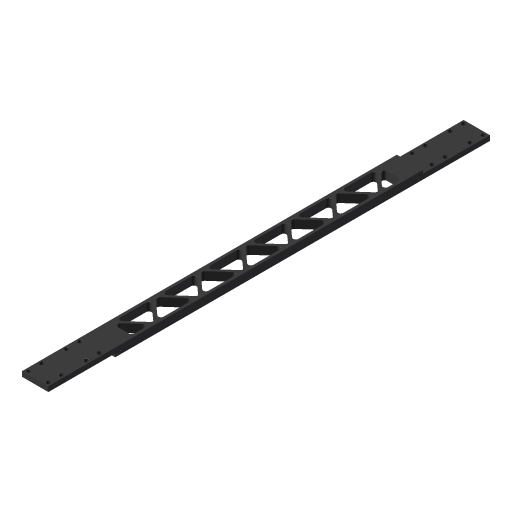
# Autodesk Inventor part: Connector Plate350mm
Saved by Autodesk Inventor 2023 (Build 270158000, 158)
## iProperties
Created: 2022-09-25
Part Number: Connector Plate350mm
Material: Generic
Document SubType Name: Modeling
Designer: deli
Density: 1 g/cm^3
Appearance: Default
Mass: 15.4529 g
Surface Area: 147.421 cm^2
Volume: 15.4529 cm^3
Author: deli
Autodesk Inventor part; units mm, degrees
ref_plane "YZ Plane" through (0, 0, 0) normal (1, 0, 0) x (0, 1, 0)
ref_plane "XZ Plane" through (0, 0, 0) normal (0, 1, 0) x (-1, 0, 0)
ref_plane "XY Plane" through (0, 0, 0) normal (0, 0, 1) x (1, 0, 0)
sketch "Sketch1" plane through (0, 0, 0) normal (0, 1, 0) x (-1, 0, 0)
  line L0 (25.6456, 366.5178) -> (5.6456, 366.5178)
  line L1 (5.6456, 366.5178) -> (5.6456, 30.4178)
  line L2 (5.6456, 30.4178) -> (25.6456, 30.4178)
  line L3 (25.6456, 30.4178) -> (25.6456, 366.5178)
  circle A0 centre (23.1456, 364.0178) radius 1.6
  circle A1 centre (23.1456, 354.0178) radius 1.6
  circle A2 centre (8.1456, 364.0178) radius 1.6
  circle A3 centre (8.1456, 354.0178) radius 1.6
  line L4 (23.1456, 364.0178) -> (23.1456, 354.0178) construction
  line L5 (23.1456, 354.0178) -> (8.1456, 354.0178) construction
  line L6 (8.1456, 354.0178) -> (8.1456, 364.0178) construction
  line L7 (8.1456, 364.0178) -> (23.1456, 364.0178) construction
  circle A4 centre (23.1456, 335.1178) radius 1.6
  circle A5 centre (23.1456, 325.1178) radius 1.6
  circle A6 centre (8.1456, 335.1178) radius 1.6
  circle A7 centre (8.1456, 325.1178) radius 1.6
  line L8 (23.1456, 335.1178) -> (23.1456, 325.1178) construction
  line L9 (23.1456, 325.1178) -> (8.1456, 325.1178) construction
  line L10 (8.1456, 325.1178) -> (8.1456, 335.1178) construction
  line L11 (8.1456, 335.1178) -> (23.1456, 335.1178) construction
  circle A8 centre (23.1456, 71.8178) radius 1.6
  circle A9 centre (23.1456, 61.8178) radius 1.6
  circle A10 centre (8.1456, 71.8178) radius 1.6
  circle A11 centre (8.1456, 61.8178) radius 1.6
  line L12 (23.1456, 71.8178) -> (23.1456, 61.8178) construction
  line L13 (23.1456, 61.8178) -> (8.1456, 61.8178) construction
  line L14 (8.1456, 61.8178) -> (8.1456, 71.8178) construction
  line L15 (8.1456, 71.8178) -> (23.1456, 71.8178) construction
  circle A12 centre (23.1456, 42.9178) radius 1.6
  circle A13 centre (23.1456, 32.9178) radius 1.6
  circle A14 centre (8.1456, 42.9178) radius 1.6
  circle A15 centre (8.1456, 32.9178) radius 1.6
  line L16 (23.1456, 42.9178) -> (23.1456, 32.9178) construction
  line L17 (23.1456, 32.9178) -> (8.1456, 32.9178) construction
  line L18 (8.1456, 32.9178) -> (8.1456, 42.9178) construction
  line L19 (8.1456, 42.9178) -> (23.1456, 42.9178) construction
  point P0 (0, 0)
  point P1 (15.6456, 30.4178)
  dimension "d0" = 20
  dimension "d23" = 3.2
  dimension "d24" = 3.2
  dimension "d25" = 3.2
  dimension "d26" = 3.2
  dimension "d27" = 15
  dimension "d28" = 10
  dimension "d29" = 2.5
  dimension "d31" = 3.2
  dimension "d32" = 3.2
  dimension "d33" = 3.2
  dimension "d34" = 3.2
  dimension "d35" = 10
  dimension "d36" = 15
  dimension "d38" = 18.9
  dimension "d49" = 10
  dimension "d50" = 15
  dimension "d58" = 10
  dimension "d59" = 15
  dimension "d63" = 18.9
  dimension "d94" = 253.3
  dimension "d101" = 331.1
  dimension "d107" = 2.5
  dimension "d108" = 2.5
  dimension "d212" = 3.2
  dimension "d213" = 2.5
  dimension "d214" = 2.5
  dimension "d215" = 2.5
  constraints: 40 end point, 16 centre point, 12 perpendicular, 7 equal radius, 4 vertical, 3 horizontal, 3 parallel, 1 midpoint
  measures "d0" distance of L2.end L1.end
  measures "d23" diameter of A0
  measures "d24" diameter of A1
  measures "d25" diameter of A2
  measures "d26" diameter of A3
  measures "d27" distance of L6.end L4.start
  measures "d28" distance of L4.start L4.end
  measures "d29" distance from line of L1 L6.end
  measures "d31" diameter of A4
  measures "d32" diameter of A5
  measures "d33" diameter of A6
  measures "d34" diameter of A7
  measures "d35" distance of L8.start L8.end
  measures "d36" distance of L10.end L8.start
  measures "d38" distance of L10.end L5.end
  measures "d49" distance of L12.end L15.end
  measures "d50" distance of L15.start L15.end
  measures "d58" distance of L19.end L16.end
  measures "d59" distance of L19.start L19.end
  measures "d63" distance of L14.start L19.start
  measures "d94" distance between parallel lines of L15 L9
  measures "d101" distance of L18.start L6.end
  measures "d107" distance from line of point (15.646, 30.418) L17
  measures "d108" distance between parallel lines of L0 L7
  measures "d212" diameter of A14
  measures "d213" distance between parallel lines of L1 L18
  measures "d214" distance between parallel lines of L1 L14
  measures "d215" distance between parallel lines of L1 L10
extrude "Extrusion1" add sketch "Sketch1" along normal blind 6.35
sketch "Sketch2" plane through (0, 6.35, 0) normal (0, 1, 0) x (1, 0, 0)
  line L0 (-5.6456, -30.4178) -> (-25.6456, -30.4178) projected
  line L1 (-5.6456, -366.5178) -> (-5.6456, -30.4178) projected
  line L2 (-25.6456, -30.4178) -> (-5.6456, -30.4178)
  line L3 (-5.6456, -30.4178) -> (-5.6456, -81.2678)
  line L4 (-5.6456, -81.2678) -> (-25.6456, -81.2678)
  line L5 (-25.6456, -81.2678) -> (-25.6456, -30.4178)
  point P0 (0, 0)
  dimension "d182" = 50.85
  constraints: 8 end point, 2 parallel, 1 horizontal, 1 perpendicular, 1 point on line
  measures "d182" distance of L2.end L3.end
extrude "Extrusion2" cut sketch "Sketch2" against normal blind 2.5
sketch "Sketch3" plane through (0, 0, 0) normal (0, -1, 0) x (1, 0, 0)
  line L0 (-25.6456, 30.4178) -> (-25.6456, 366.5178) projected
  line L1 (-5.6456, 366.5178) -> (-5.6456, 30.4178) projected
  line L2 (-25.6456, 366.5178) -> (-5.6456, 366.5178)
  line L3 (-5.6456, 366.5178) -> (-5.6456, 315.6678)
  line L4 (-5.6456, 315.6678) -> (-25.6456, 315.6678)
  line L5 (-25.6456, 315.6678) -> (-25.6456, 366.5178)
  point P0 (0, 0)
  point P1 (-5.6456, 366.5178)
  point P2 (-25.6456, 315.6678)
  dimension "d192" = 50.85
  constraints: 8 end point, 2 parallel, 1 horizontal, 1 perpendicular, 1 point on line
  measures "d192" distance of L2.end L3.end
extrude "Extrusion3" cut sketch "Sketch3" against normal blind 2.5
sketch "Sketch4" plane through (-5.6456, 6.35, 366.5178) normal (1, 0, 0) x (0, 0, -1)
  circle A0 centre (282, -3.175) radius 1.25
  line L0 (50.85, -6.35) -> (336.1, -6.35) projected
  line L1 (285.25, -2.5) -> (285.25, 0) projected
  circle A1 centre (54.1, -3.175) radius 1.25
  line L2 (50.85, -3.85) -> (50.85, -6.35) projected
  point P0 (366.5178, -6.35)
  dimension "d196" = 2.5
  dimension "d199" = 2
  dimension "d200" = 3.175
  dimension "d207" = 2.5
  dimension "d208" = 2
  dimension "d209" = 3.175
  constraints: 2 centre point
  measures "d196" diameter of A0
  measures "d199" distance edge to line of A0 L1
  measures "d200" distance from line of L0 A0.centre
  measures "d207" diameter of A1
  measures "d208" distance edge to line of A1 L2
  measures "d209" distance from line of A1.centre L0
extrude "Extrusion4" cut sketch "Sketch4" against normal blind 8
thread "Thread1" size "M3x0.5" class "6H" standard "ANSI Metric M Profile" full length
thread "Thread3" size "M3x0.5" class "6H" standard "ANSI Metric M Profile" full length
sketch "Sketch5" plane through (0, 6.35, 0) normal (0, 1, 0) x (1, 0, 0)
  line L0 (-5.6456, -81.2678) -> (-25.6456, -81.2678) projected
  line L1 (-5.6456, -315.6678) -> (-25.6456, -315.6678) projected
  line L2 (-25.6456, -315.6678) -> (-25.6456, -81.2678)
  line L3 (-5.6456, -81.2678) -> (-5.6456, -315.6678)
  line L4 (-23.6456, -98.5726) -> (-23.6456, -127.3856)
  line L5 (-23.6456, -127.3856) -> (-7.6456, -112.9791)
  line L6 (-7.6456, -112.9791) -> (-23.6456, -98.5726)
  line L7 (-23.6456, -95.8814) -> (-7.6456, -95.8814)
  line L8 (-7.6456, -95.8814) -> (-7.6456, -110.2878)
  line L9 (-7.6456, -110.2878) -> (-23.6456, -95.8814)
  line L10 (-7.6456, -115.6704) -> (-23.6456, -130.0768)
  line L11 (-23.6456, -130.0768) -> (-7.6456, -144.4833)
  line L12 (-7.6456, -144.4833) -> (-7.6456, -115.6704)
  line L13 (-23.6456, -132.7681) -> (-7.6456, -147.1746)
  line L14 (-7.6456, -147.1746) -> (-23.6456, -161.581)
  line L15 (-23.6456, -161.581) -> (-23.6456, -132.7681)
  line L16 (-7.6456, -149.8658) -> (-23.6456, -164.2723)
  line L17 (-23.6456, -164.2723) -> (-7.6456, -178.6788)
  line L18 (-7.6456, -178.6788) -> (-7.6456, -149.8658)
  line L19 (-23.6456, -166.9636) -> (-7.6456, -181.37)
  line L20 (-7.6456, -181.37) -> (-23.6456, -195.7765)
  line L21 (-23.6456, -195.7765) -> (-23.6456, -166.9636)
  line L22 (-7.6456, -184.0613) -> (-23.6456, -198.4678)
  line L23 (-23.6456, -198.4678) -> (-7.6456, -212.8742)
  line L24 (-7.6456, -212.8742) -> (-7.6456, -184.0613)
  line L25 (-23.6456, -201.159) -> (-23.6456, -229.972)
  line L26 (-23.6456, -229.972) -> (-7.6456, -215.5655)
  line L27 (-7.6456, -215.5655) -> (-23.6456, -201.159)
  line L28 (-7.6456, -218.2568) -> (-23.6456, -232.6632)
  line L29 (-23.6456, -232.6632) -> (-7.6456, -247.0697)
  line L30 (-7.6456, -247.0697) -> (-7.6456, -218.2568)
  line L31 (-23.6456, -235.3545) -> (-7.6456, -249.761)
  line L32 (-7.6456, -249.761) -> (-23.6456, -264.1674)
  line L33 (-23.6456, -264.1674) -> (-23.6456, -235.3545)
  line L34 (-23.6456, -301.0541) -> (-7.6456, -286.6477)
  line L35 (-23.6456, -301.0541) -> (-7.6456, -301.0541)
  line L36 (-7.6456, -286.6477) -> (-7.6456, -301.0541)
  line L37 (-7.6456, -252.4522) -> (-7.6456, -281.2651)
  line L38 (-7.6456, -281.2651) -> (-23.6456, -266.8587)
  line L39 (-23.6456, -266.8587) -> (-7.6456, -252.4522)
  line L40 (-23.6456, -269.5499) -> (-23.6456, -298.3629)
  line L41 (-23.6456, -298.3629) -> (-7.6456, -283.9564)
  line L42 (-7.6456, -283.9564) -> (-23.6456, -269.5499)
  point P0 (0, 0)
  dimension "d107" = 2.5
  dimension "d216" = 48
  dimension "d217" = 2
  dimension "d218" = 2
  dimension "d221" = 2
  dimension "d227" = 2
  dimension "d228" = 2
  dimension "d232" = 2
  dimension "d233" = 2
  dimension "d234" = 234.4
  dimension "d235" = 2
  dimension "d236" = 2
  dimension "d237" = 2
  dimension "d238" = 2
  dimension "d244" = 2
  dimension "d245" = 2
  dimension "d246" = 2
  dimension "d248" = 205.1728
  dimension "d249" = 14.6136
  constraints: 82 end point, 25 parallel, 19 point on line, 10 equal length, 4 collinear, 4 vertical, 3 perpendicular, 1 horizontal
  measures "d216" angle of L6 L4
  measures "d217" distance between parallel lines of L2 L4
  measures "d218" distance between parallel lines of L3 L8
  measures "d221" distance from line of L6 L7.start
  measures "d227" distance between parallel lines of L10 L5
  measures "d228" distance between parallel lines of L11 L13
  measures "d232" distance between parallel lines of L16 L14
  measures "d233" distance between parallel lines of L17 L19
  measures "d234" distance between parallel lines of L1 L0
  measures "d235" distance between parallel lines of L22 L20
  measures "d236" distance between parallel lines of L23 L27
  measures "d237" distance between parallel lines of L28 L26
  measures "d238" distance between parallel lines of L29 L31
  measures "d244" distance between parallel lines of L39 L32
  measures "d245" distance between parallel lines of L38 L42
  measures "d246" distance between parallel lines of L34 L41
  measures "d248" distance between parallel lines of L7 L35
  measures "d249" distance between parallel lines of L0 L7
extrude "Extrusion5" cut sketch "Sketch5" against normal blind 10 contours L6 L5 L4 | L7 L8 L9 | L12 L11 L10 | L13 L14 L15 | L18 L17 L16 | L19 L20 L21 | L24 L23 L22 | L27 L26 L25 | L30 L29 L28 | L31 L32 L33 | L34 L36 L35 | L37 L38 L39 | L42 L41 L40
fillet "Fillet3" radius 2 39 edges at (-7.6456, 3.175, 301.0541) (-23.6456, 3.175, 301.0541) (-7.6456, 3.175, 286.6477) (-23.6456, 3.175, 264.1674) (-7.6456, 3.175, 249.761) (-23.6456, 3.175, 235.3545) (-23.6456, 3.175, 232.6632) (-7.6456, 3.175, 247.0697) (-7.6456, 3.175, 218.2568) (-23.6456, 3.175, 229.972) (-7.6456, 3.175, 215.5655) (-23.6456, 3.175, 201.159) (-23.6456, 3.175, 198.4678) (-7.6456, 3.175, 212.8742) (-7.6456, 3.175, 184.0613) (-23.6456, 3.175, 195.7765) (-7.6456, 3.175, 181.37) (-23.6456, 3.175, 166.9636) (-23.6456, 3.175, 164.2723) (-23.6456, 3.175, 161.581) (-7.6456, 3.175, 178.6788) (-7.6456, 3.175, 149.8658) (-7.6456, 3.175, 147.1746) (-7.6456, 3.175, 144.4833) (-23.6456, 3.175, 132.7681) (-23.6456, 3.175, 130.0768) (-23.6456, 3.175, 127.3856) (-7.6456, 3.175, 115.6704) (-7.6456, 3.175, 112.9791) (-7.6456, 3.175, 110.2878) (-23.6456, 3.175, 98.5726) (-23.6456, 3.175, 95.8814) (-7.6456, 3.175, 95.8814) (-23.6456, 3.175, 269.5499) (-7.6456, 3.175, 281.2651) (-23.6456, 3.175, 266.8587) (-7.6456, 3.175, 252.4522) (-7.6456, 3.175, 283.9564) (-23.6456, 3.175, 298.3629)
equation "\"d24\" = d23"
equation "\"d25\" = d23"
equation "\"d26\" = d23"
equation "\"d29\" = -0.5 * d27 + 0.5 * d0"
equation "\"d31\" = d23"
equation "\"d32\" = d23"
equation "\"d33\" = d23"
equation "\"d34\" = d23"
equation "\"d35\" = d28"
equation "\"d36\" = d27"
equation "\"d49\" = d52"
equation "\"d50\" = d53"
equation "\"d58\" = d61"
equation "\"d59\" = d62"
equation "\"d63\" = d38"
equation "\"d52\" = 10"
equation "\"d53\" = 15"
equation "\"d61\" = 10"
equation "\"d62\" = 15"
body "Solid1"
